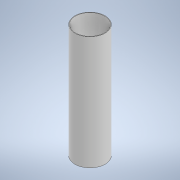
# Autodesk Inventor part: 回收桶
Saved by Autodesk Inventor 2020 (Build 240168000, 168)
## iProperties
Created: 2020-12-03
Part Number: 回收桶
Material: 常规
Document SubType Name: Sheet Metal
Designer: huang
Density: 1 g/cm^3
Sheet Metal Rule: 默认_mm
Appearance: 默认
Author: huang
Autodesk Inventor part; units mm, degrees
ref_plane "YZ Plane" through (0, 0, 0) normal (1, 0, 0) x (0, 1, 0)
ref_plane "XZ Plane" through (0, 0, 0) normal (0, 1, 0) x (-1, 0, 0)
ref_plane "XY Plane" through (0, 0, 0) normal (0, 0, 1) x (1, 0, 0)
sketch "草图1" plane through (0, 0, 0) normal (0, 1, 0) x (-1, 0, 0)
  circle A0 centre (0, 0) radius 40
  circle A1 centre (0, 0) radius 38.5
  dimension "d0" = 80
  dimension "d1" = 77
  constraints: 2 centre point, 2 coincident
  measures "d0" diameter of A0
  measures "d1" diameter of A1
extrude "拉伸1" add sketch "草图1" along normal blind 300
sketch "草图9" plane through (0, 0, 0) normal (1, 0, 0) x (0, 1, 0)
  circle A0 centre (18.9064, 0) radius 1.5
  point P0 (0, 0)
  dimension "d14" = 3
  constraints: 1 centre point
  measures "d14" diameter of A0
extrude "拉伸5" cut sketch "草图9" against normal blind 300
equation "\"折弯半径\" = 厚度"
equation "\"折弯释压宽度\" = 厚度"
equation "\"折弯释压深度\" = 0.5 * 厚度"
equation "\"拐角释压尺寸\" = 4 * 厚度"
equation "\"最小余量\" = 2 * 厚度"
equation "\"过渡半径\" = 折弯半径"
equation "\"Jacobi半径尺寸\" = 折弯半径"
equation "\"间隙大小\" = 厚度"
equation "\"厚度\" = 0.5"
